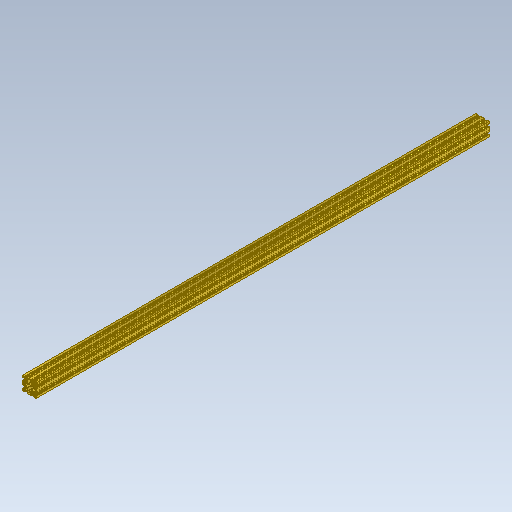
# Autodesk Inventor part: Perfil 60×60 8 rasgos_AST06006008
Saved by Autodesk Inventor 2025.2 (Build 292293000, 293)
## iProperties
Created: 2025-04-07
Part Number: Perfil 60×60 8 rasgos_AST06006008
Material: Ouro
Document SubType Name: Modeling
Designer: Gustavo Sousa
Density: 19.3 g/cm^3
Appearance: Metal quente 2400F
Author: Gustavo Sousa
Autodesk Inventor part; units mm, degrees
ref_plane "YZ Plane" through (0, 0, 0) normal (1, 0, 0) x (0, 1, 0)
ref_plane "XZ Plane" through (0, 0, 0) normal (0, 1, 0) x (-1, 0, 0)
ref_plane "XY Plane" through (0, 0, 0) normal (0, 0, 1) x (1, 0, 0)
sketch "Esboço1" plane through (0, 0, 0) normal (0, 0, 1) x (1, 0, 0)
  line L0 (-30, 30) -> (30, 30) construction
  line L1 (-30, 30) -> (-30, -30) construction
  circle A0 centre (-15, 15) radius 5
  line L2 (-30, 30) -> (0, 30) construction
  line L3 (-22, 22) -> (-8, 22) construction
  line L4 (-19.1, 30) -> (-10.9, 30)
  line L5 (-15, 15) -> (-30, 30) construction
  line L6 (-22, 22) -> (-22, 8) construction
  line L7 (-19.1, 30) -> (-19.6, 30) construction
  line L8 (-19.6, 30) -> (-19.6, 29.5)
  line L9 (-19.6, 29.5) -> (-19.1, 29.5)
  line L10 (-19.1, 29.5) -> (-19.1, 30) construction
  arc A1 (-29.5, 30) -> (-30, 29.5) centre (-29.5, 29.5) ccw
  line L11 (-29.5, 30) -> (-19.6, 30)
  line L12 (-23.15, 24.7056) -> (-20.4444, 22) construction
  line L13 (-19.1, 30) -> (-19.1, 27.8) construction
  line L14 (-19.1, 27.8) -> (-23.15, 27.8) construction
  line L15 (-19.1, 29.5) -> (-19.1, 27.8)
  line L16 (-23.15, 24.7056) -> (-23.15, 27.8) construction
  line L17 (-20.4444, 22) -> (-15, 22) construction
  circle A2 centre (-26.5, 26.5) radius 2.25
  line L18 (-10.9, 30) -> (-10.4, 30) construction
  line L19 (-10.4, 30) -> (-10.4, 29.5)
  line L20 (-10.4, 29.5) -> (-10.9, 29.5)
  line L21 (-10.9, 29.5) -> (-10.9, 30) construction
  line L22 (-10.4, 30) -> (0, 30)
  line L23 (-15, 15) -> (0, 30) construction
  line L24 (-8, 22) -> (-8, 8) construction
  line L25 (-10.9, 30) -> (-10.9, 27.8) construction
  line L26 (-10.9, 27.8) -> (-6.85, 27.8) construction
  line L27 (-10.9, 29.5) -> (-10.9, 27.8)
  line L28 (-9.5556, 22) -> (-6.85, 24.7056) construction
  line L29 (-6.85, 27.8) -> (-6.85, 24.7056) construction
  line L30 (-15, 22) -> (-9.5556, 22) construction
  line L31 (0, 30) -> (0, 27.8)
  line L32 (0, 27.8) -> (-4.65, 27.8) construction
  line L33 (-8, 20.4444) -> (-4.65, 23.7944) construction
  line L34 (-4.65, 27.8) -> (-4.65, 23.7944) construction
  line L35 (-30, 30) -> (-30, 0) construction
  line L36 (-30, 19.1) -> (-30, 10.9) construction
  line L37 (-15, 15) -> (-30, 0) construction
  line L38 (-8, 8) -> (-22, 8) construction
  line L39 (-30, 19.1) -> (-29.5, 19.1) construction
  line L40 (-29.5, 19.1) -> (-29.5, 19.6)
  line L41 (-29.5, 19.6) -> (-30, 19.6)
  line L42 (-30, 19.6) -> (-30, 19.1) construction
  line L43 (-30, 19.6) -> (-30, 29.5)
  line L44 (-30, 19.1) -> (-27.8, 19.1) construction
  line L45 (-27.8, 19.1) -> (-27.8, 23.15) construction
  line L46 (-24.7056, 23.15) -> (-22, 20.4444) construction
  line L47 (-27.8, 23.15) -> (-24.7056, 23.15) construction
  line L48 (-29.5, 19.1) -> (-27.8, 19.1)
  line L49 (-27.8, 19.1) -> (-27.8, 23.15) construction
  line L50 (-27.8, 23.15) -> (-24.7056, 23.15) construction
  line L51 (-22, 20.4444) -> (-22, 15) construction
  line L52 (-30, 10.9) -> (-29.5, 10.9) construction
  line L53 (-29.5, 10.9) -> (-29.5, 10.4)
  line L54 (-29.5, 10.4) -> (-30, 10.4)
  line L55 (-30, 10.4) -> (-30, 10.9) construction
  line L56 (-30, 10.9) -> (-27.8, 10.9) construction
  line L57 (-27.8, 10.9) -> (-27.8, 6.85) construction
  line L58 (-27.8, 6.85) -> (-24.7056, 6.85) construction
  line L59 (-22, 9.5556) -> (-24.7056, 6.85) construction
  line L60 (-22, 9.5556) -> (-22, 15) construction
  line L61 (-29.5, 10.9) -> (-27.8, 10.9)
  line L62 (-30, 10.4) -> (-30, 0)
  line L63 (-23.7944, 4.65) -> (-20.4444, 8) construction
  line L64 (-23.7944, 4.65) -> (-27.8, 4.65) construction
  line L65 (-30, 0) -> (-27.8, 0)
  line L66 (-27.8, 0) -> (-27.8, 4.65) construction
  line L67 (-20.4444, 8) -> (-8, 8) construction
  line L68 (-8, 8) -> (-8, 20.4444) construction
  circle A3 centre (-18.5355, 18.5355) radius 1.1
  circle A4 centre (-18.5355, 11.4645) radius 1.1
  circle A5 centre (-11.4645, 11.4645) radius 1.1
  circle A6 centre (-11.4645, 18.5355) radius 1.1
  arc A7 (-20.5908, 22.1464) -> (-20.2373, 22) centre (-20.2373, 22.5) ccw
  arc A8 (-23.15, 24.9127) -> (-23.0036, 24.5592) centre (-22.65, 24.9127) ccw
  arc A9 (-22.65, 27.8) -> (-23.15, 27.3) centre (-22.65, 27.3) ccw
  arc A10 (-6.85, 27.3) -> (-7.35, 27.8) centre (-7.35, 27.3) ccw
  arc A11 (-6.9964, 24.5592) -> (-6.85, 24.9127) centre (-7.35, 24.9127) ccw
  arc A12 (-9.7627, 22) -> (-9.4092, 22.1464) centre (-9.7627, 22.5) ccw
  line L69 (-22.65, 27.8) -> (-19.1, 27.8)
  line L70 (-10.9, 27.8) -> (-7.35, 27.8)
  line L71 (-6.85, 27.3) -> (-6.85, 24.9127)
  line L72 (-6.9964, 24.5592) -> (-9.4092, 22.1464)
  line L73 (-23.15, 27.3) -> (-23.15, 24.9127)
  line L74 (-23.0036, 24.5592) -> (-20.5908, 22.1464)
  line L75 (-20.2373, 22) -> (-15, 22)
  line L76 (-9.7627, 22) -> (-15, 22)
  arc A13 (-4.15, 27.8) -> (-4.65, 27.3) centre (-4.15, 27.3) ccw
  arc A14 (-4.7964, 23.6479) -> (-4.65, 24.0015) centre (-5.15, 24.0015) ccw
  arc A15 (-7.8536, 20.5908) -> (-8, 20.2373) centre (-7.5, 20.2373) ccw
  arc A16 (-8.5, 8) -> (-8, 8.5) centre (-8.5, 8.5) ccw
  line L77 (-4.15, 27.8) -> (0, 27.8)
  line L78 (-4.65, 27.3) -> (-4.65, 24.0015)
  line L79 (-4.7964, 23.6479) -> (-7.8536, 20.5908)
  line L80 (-8, 20.2373) -> (-8, 8.5)
  arc A17 (-20.2373, 8) -> (-20.5908, 7.8536) centre (-20.2373, 7.5) ccw
  arc A18 (-24.0015, 4.65) -> (-23.6479, 4.7964) centre (-24.0015, 5.15) ccw
  arc A19 (-27.3, 4.65) -> (-27.8, 4.15) centre (-27.3, 4.15) ccw
  line L81 (-20.2373, 8) -> (-8.5, 8)
  line L82 (-20.5908, 7.8536) -> (-23.6479, 4.7964)
  line L83 (-24.0015, 4.65) -> (-27.3, 4.65)
  line L84 (-27.8, 4.15) -> (-27.8, 0)
  arc A20 (-27.3, 23.15) -> (-27.8, 22.65) centre (-27.3, 22.65) ccw
  arc A21 (-24.5592, 23.0036) -> (-24.9127, 23.15) centre (-24.9127, 22.65) ccw
  arc A22 (-22, 20.2373) -> (-22.1464, 20.5908) centre (-22.5, 20.2373) ccw
  arc A23 (-22.1464, 9.4092) -> (-22, 9.7627) centre (-22.5, 9.7627) ccw
  arc A24 (-24.9127, 6.85) -> (-24.5592, 6.9964) centre (-24.9127, 7.35) ccw
  arc A25 (-27.8, 7.35) -> (-27.3, 6.85) centre (-27.3, 7.35) ccw
  line L85 (-27.8, 22.65) -> (-27.8, 19.1)
  line L86 (-27.3, 23.15) -> (-24.9127, 23.15)
  line L87 (-24.5592, 23.0036) -> (-22.1464, 20.5908)
  line L88 (-27.8, 10.9) -> (-27.8, 7.35)
  line L89 (-27.3, 6.85) -> (-24.9127, 6.85)
  line L90 (-24.5592, 6.9964) -> (-22.1464, 9.4092)
  line L91 (-22, 9.7627) -> (-22, 15)
  line L92 (-22, 20.2373) -> (-22, 15)
  point P0 (0, 0)
  point P1 (-15, 30)
  point P2 (-15, 30)
  point P3 (-30, 15)
  point P4 (-30, 15)
  point P5 (-12.3231, 19.2231)
  point P6 (-10.7769, 17.6769)
  point P7 (-10.7769, 12.3231)
  point P8 (-12.3231, 10.7769)
  point P9 (-17.6769, 10.7769)
  point P10 (-19.2231, 12.3231)
  point P11 (-19.2231, 17.6769)
  point P12 (-17.6769, 19.2231)
  dimension "d5" = 10
  dimension "d0" = 30
  dimension "d1" = 60
  dimension "d3" = 15
  dimension "d4" = 15
  dimension "d6" = 8
  dimension "d7" = 8.2
  dimension "d8" = 0.5
  dimension "d9" = 0.5
  dimension "d10" = 1.1
  dimension "d12" = 2.2
  dimension "d14" = 26.5
  dimension "d15" = 4.5
  dimension "d16" = 1.1
  dimension "d18" = 2.2
  dimension "d19" = 1.1
  dimension "d21" = 2.2
  dimension "d24" = 360
  constraints: 186 end point, 49 point on line, 42 tangent, 40 point on circle, 33 collinear, 25 centre point, 20 equal length, 19 equal radius, 16 horizontal, 14 parallel, 11 perpendicular, 11 vertical, 8 midpoint, 4 coincident, 4 vertical alignment, 2 horizontal alignment, 12 other
  measures "d0" distance from line of point (0, 0) L0
  measures "d1" distance of L0.start L0.end
  measures "d3" horizontal distance of point (0, 0) L5.start
  measures "d4" horizontal distance of point (0, 0) L5.start
  measures "d6" distance between parallel lines of L0 L3
  measures "d7" distance of L4.start L4.end
  measures "d8" distance of L9.end L4.start
  measures "d9" radius of A1
  measures "d10" distance between parallel lines of L5 L12
  measures "d12" distance between parallel lines of L0 L14
  measures "d14" horizontal distance of point (0, 0) A2.centre
  measures "d15" diameter of A2
  measures "d16" distance edge to line of A2 L16
  measures "d18" distance of L32.end L26.end
  measures "d19" distance between parallel lines of L23 L33
  measures "d21" diameter of A3
extrude "Extrusão1" add sketch "Esboço1" along normal mid plane 2000
mirror "Espelhar1" about plane through (0, 0, 0) normal (0, 1, 0) of "Extrusão1"
mirror "Espelhar2" about plane through (0, 0, 0) normal (1, 0, 0) of "Extrusão1", "Espelhar1"
